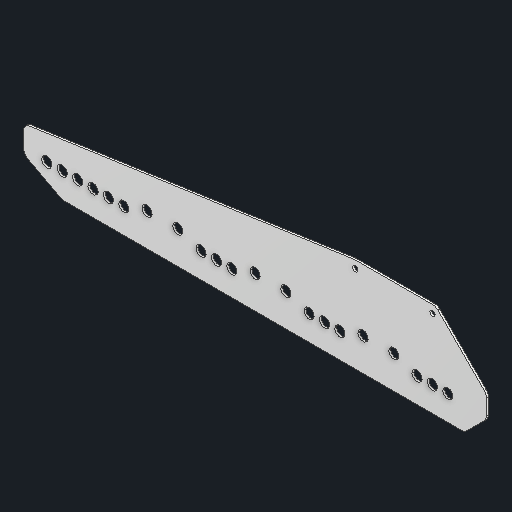
# Autodesk Inventor part: skirt
Saved by Autodesk Inventor 2025 (Build 290162000, 162)
## iProperties
Created: 2024-10-14
Part Number: skirt
Material: Acetal Resin, White
Document SubType Name: Modeling
Designer: Averey Ku
Density: 1.425 g/cm^3
Appearance: Smooth - White
Author: Averey Ku
Autodesk Inventor part; units mm, degrees
ref_plane "YZ Plane" through (0, 0, 0) normal (1, 0, 0) x (0, 1, 0)
ref_plane "XZ Plane" through (0, 0, 0) normal (0, 1, 0) x (-1, 0, 0)
ref_plane "XY Plane" through (0, 0, 0) normal (0, 0, 1) x (1, 0, 0)
sketch "main" plane through (0, 0, 0) normal (0, 0, 1) x (1, 0, 0)
  circle A0 centre (-13.3607, 90.7974) radius 2.1844
  circle A1 centre (-19.7107, 109.8474) radius 2.1844
  circle A2 centre (-19.7107, 122.5474) radius 2.1358
  circle A3 centre (-19.7107, 147.9474) radius 2.1844
  circle A4 centre (-19.7107, 135.2474) radius 2.1844
  circle A5 centre (-19.7107, 173.3474) radius 2.1844
  circle A6 centre (-19.7107, 160.6474) radius 2.1844
  circle A7 centre (-13.3607, 65.3974) radius 2.1844
  circle A8 centre (-19.7107, 46.3474) radius 2.1844
  circle A9 centre (-19.7107, 33.6474) radius 2.1844
  circle A10 centre (-19.7107, 20.9474) radius 2.1844 construction
  line L0 (-1.5114, 189.2224) -> (37.374, -79.744)
  line L1 (-40.3482, -167.9651) -> (-40.3482, 159.8585)
  circle A11 centre (-13.3607, 1.8974) radius 2.1844 construction
  circle A12 centre (-13.3607, -23.5026) radius 2.1844 construction
  circle A13 centre (-19.7107, -42.5526) radius 2.1844 construction
  circle A14 centre (-19.7107, -67.9526) radius 2.1844 construction
  circle A15 centre (31.0893, -80.6526) radius 2.1844
  circle A16 centre (-19.7107, -55.2526) radius 2.1844 construction
  circle A17 centre (-13.3607, -87.0026) radius 2.1844 construction
  circle A18 centre (-13.3607, -112.4026) radius 2.1844 construction
  circle A19 centre (-19.7107, -131.4526) radius 2.1844 construction
  circle A20 centre (-19.7107, -144.1526) radius 2.1844 construction
  line L2 (37.374, -79.744) -> (37.4393, -144.1462)
  arc A21 (35.5805, -148.6417) -> (37.4393, -144.1462) centre (31.0893, -144.1526) ccw
  arc A22 (37.3758, -81.5485) -> (37.374, -79.744) centre (31.0893, -80.6526) ccw
  circle A23 centre (-19.7107, -156.8526) radius 2.1844 construction
  arc A24 (-40.3482, -167.9651) -> (-38.4883, -172.4553) centre (-33.9982, -167.9651) ccw
  line L3 (35.5805, -148.6417) -> (-2.5106, -186.7506)
  line L4 (-2.5106, -186.7506) -> (-1.346, -186.7506) construction
  arc A25 (-7.3374, -188.6026) -> (-2.5106, -186.7506) centre (-7.0018, -182.2615) ccw
  line L5 (-24.1929, -186.7506) -> (-38.4883, -172.4553)
  line L6 (-7.3374, -188.6026) -> (-19.7047, -188.6066)
  arc A26 (-24.2008, -186.7428) -> (-19.7047, -188.6066) centre (-19.7067, -182.2566) ccw
  circle A27 centre (31.0893, -144.1526) radius 2.1844
  arc A28 (-19.7107, 192.3974) -> (-25.3223, 189.0193) centre (-19.7107, 186.0474) ccw
  arc A29 (-0.8373, 184.5599) -> (-7.0107, 192.3974) centre (-7.0107, 186.0474) ccw
  arc A30 (-39.979, 161.3445) -> (-40.3482, 159.8585) centre (-37.1732, 159.8585) ccw
  line L7 (-39.979, 161.3445) -> (-25.3223, 189.0193)
  line L8 (-19.7107, 192.3974) -> (-7.0107, 192.3974)
  circle A31 centre (-19.7107, 173.3474) radius 4.2164
  circle A32 centre (-19.7107, 160.6474) radius 4.2166
  circle A33 centre (-19.7107, 147.9474) radius 4.2167
  circle A34 centre (-19.7107, 135.2474) radius 4.2169
  circle A35 centre (-19.7107, 122.5474) radius 4.217
  circle A36 centre (-19.7107, 109.8474) radius 4.2171
  circle A37 centre (-13.3607, 90.7974) radius 4.2164
  circle A38 centre (-13.3607, 65.3974) radius 4.2167
  circle A39 centre (-19.7107, 46.3474) radius 4.2178
  circle A40 centre (-19.7107, 33.6474) radius 4.2179
  circle A41 centre (-19.7107, 20.9474) radius 4.2181
  circle A42 centre (-13.3607, 1.8974) radius 4.2173
  circle A43 centre (-13.3607, -23.5026) radius 4.2176
  circle A44 centre (-19.7107, -42.5526) radius 4.2188
  circle A45 centre (-19.7107, -55.2526) radius 4.2189
  circle A46 centre (-19.7107, -67.9526) radius 4.219
  circle A47 centre (-13.3607, -87.0026) radius 4.2183
  circle A48 centre (-13.3607, -112.4026) radius 4.2186
  circle A49 centre (-19.7107, -131.4526) radius 4.2197
  circle A50 centre (-19.7107, -144.1526) radius 4.2198
  circle A51 centre (-19.7107, -156.8526) radius 4.22
  point P0 (-9.7209, -19.0127)
  dimension "d0" = 135
  dimension "d1" = 135
  dimension "d2" = 6.35
  dimension "d3" = 3.175
  dimension "d4" = 8.4328
  dimension "d5" = 8.4328
  measures "d0" angle of L4 L5
  measures "d1" angle of L5 L1
  measures "d2" radius of A24
  measures "d3" radius of A30
  measures "d4" diameter of A31
  measures "d5" diameter of A37
sketch "Sketch1" plane through (0, 0, 0) normal (0, 0, 1) x (1, 0, 0)
  circle A0 centre (95.2501, 6.349) radius 2.1844
  circle A1 centre (76.2, -0.0008) radius 2.1844
  circle A2 centre (63.5, -0.0007) radius 2.1358
  circle A3 centre (38.1, -0.0004) radius 2.1844
  circle A4 centre (50.8, -0.0005) radius 2.1844
  circle A5 centre (12.7, -0.0001) radius 2.1844
  circle A6 centre (25.4, -0.0003) radius 2.1844
  circle A7 centre (120.6501, 6.3487) radius 2.1844
  circle A8 centre (139.7, -0.0015) radius 2.1844
  circle A9 centre (152.4, -0.0016) radius 2.1844
  circle A10 centre (165.1, -0.0018) radius 2.1844 construction
  line L0 (-3.1748, 18.1993) -> (265.792, 57.0818)
  line L1 (354.0123, -20.6413) -> (26.1886, -20.6378)
  circle A11 centre (184.1501, 6.348) radius 2.1844 construction
  circle A12 centre (209.5501, 6.3478) radius 2.1844 construction
  circle A13 centre (228.6, -0.0024) radius 2.1844 construction
  circle A14 centre (254, -0.0027) radius 2.1844 construction
  circle A15 centre (266.7005, 50.7972) radius 2.1844
  circle A16 centre (241.3, -0.0026) radius 2.1844 construction
  circle A17 centre (273.0501, 6.3471) radius 2.1844 construction
  circle A18 centre (298.4501, 6.3468) radius 2.1844 construction
  circle A19 centre (317.5, -0.0034) radius 2.1844 construction
  circle A20 centre (330.2, -0.0035) radius 2.1844 construction
  line L2 (265.792, 57.0818) -> (330.1942, 57.1465)
  arc A21 (334.6897, 55.2876) -> (330.1942, 57.1465) centre (330.2005, 50.7965) ccw
  arc A22 (267.5964, 57.0836) -> (265.792, 57.0818) centre (266.7005, 50.7972) ccw
  circle A23 centre (342.9, -0.0036) radius 2.1844 construction
  arc A24 (354.0123, -20.6413) -> (358.5024, -18.7814) centre (354.0123, -14.2913) ccw
  line L3 (334.6897, 55.2876) -> (372.7981, 17.1961)
  line L4 (372.7981, 17.1961) -> (372.7982, 18.3607) construction
  arc A25 (374.6501, 12.3693) -> (372.7981, 17.1961) centre (368.309, 12.705) ccw
  line L5 (372.7979, -4.4862) -> (358.5024, -18.7814)
  line L6 (374.6501, 12.3693) -> (374.6539, 0.0019)
  arc A26 (372.7901, -4.4941) -> (374.6539, 0.0019) centre (368.3039, 0) ccw
  circle A27 centre (330.2005, 50.7965) radius 2.1844
  arc A28 (-6.35, 0.0001) -> (-2.972, -5.6116) centre (0, 0) ccw
  arc A29 (1.4877, 18.8733) -> (-6.3499, 12.7001) centre (0.0001, 12.7) ccw
  arc A30 (24.7027, -20.2686) -> (26.1886, -20.6378) centre (26.1887, -17.4628) ccw
  line L7 (24.7027, -20.2686) -> (-2.972, -5.6116)
  line L8 (-6.35, 0.0001) -> (-6.3499, 12.7001)
  circle A31 centre (12.7, -0.0001) radius 4.2164
  circle A32 centre (25.4, -0.0003) radius 4.2166
  circle A33 centre (38.1, -0.0004) radius 4.2167
  circle A34 centre (50.8, -0.0005) radius 4.2169
  circle A35 centre (63.5, -0.0007) radius 4.217
  circle A36 centre (76.2, -0.0008) radius 4.2171
  circle A37 centre (95.2501, 6.349) radius 4.2164
  circle A38 centre (120.6501, 6.3487) radius 4.2167
  circle A39 centre (139.7, -0.0015) radius 4.2178
  circle A40 centre (152.4, -0.0016) radius 4.2179
  circle A41 centre (165.1, -0.0018) radius 4.2181
  circle A42 centre (184.1501, 6.348) radius 4.2173
  circle A43 centre (209.5501, 6.3478) radius 4.2176
  circle A44 centre (228.6, -0.0024) radius 4.2188
  circle A45 centre (241.3, -0.0026) radius 4.2189
  circle A46 centre (254, -0.0027) radius 4.219
  circle A47 centre (273.0501, 6.3471) radius 4.2183
  circle A48 centre (298.4501, 6.3468) radius 4.2186
  circle A49 centre (317.5, -0.0034) radius 4.2197
  circle A50 centre (330.2, -0.0035) radius 4.2198
  circle A51 centre (342.9, -0.0036) radius 4.22
  point P0 (0, 0)
  constraints: 1 other
extrude "Extrusion1" add sketch "Sketch1" along normal blind 1.5875 contours L0 L2 A21 L3 A25 L6 A26 L5 A24 L1 A30 L7 A28 L8 A29
body "Solid1"
